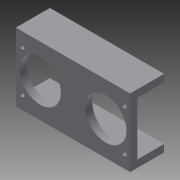
# Autodesk Inventor part: ProxSensor_Bracket
Saved by Autodesk Inventor 2015 (Build 190159000, 159)
## iProperties
Created: 2015-03-05
Part Number: ProxSensor_Bracket
Material: Generic
Document SubType Name: Modeling
Designer: ChristopherEvan
Density: 1 g/cm^3
Appearance: Default
Author: ChristopherEvan
Autodesk Inventor part; units mm, degrees
ref_plane "YZ Plane" through (0, 0, 0) normal (1, 0, 0) x (0, 1, 0)
ref_plane "XZ Plane" through (0, 0, 0) normal (0, 1, 0) x (-1, 0, 0)
ref_plane "XY Plane" through (0, 0, 0) normal (0, 0, 1) x (1, 0, 0)
sketch "Sketch1" plane through (0, 0, 0) normal (0, 0, 1) x (1, 0, 0)
  circle A0 centre (36, -10) radius 0.8353 projected
  circle A1 centre (9, -10) radius 0.8353 projected
  circle A2 centre (1.5, -1.5) radius 1 projected
  circle A3 centre (1.5, -18.5) radius 1 projected
  circle A4 centre (43.5, -1.5) radius 1 projected
  circle A5 centre (43.5, -18.5) radius 1 projected
  line L0 (0, -20) -> (45, -20) projected
  line L1 (45, -20) -> (45, 0) projected
  line L2 (45, 0) -> (0, 0) projected
  line L3 (0, 0) -> (0, -20) projected
  circle A6 centre (36, -10) radius 8.5
  line L4 (46, 1) -> (-1, 1)
  line L5 (-1, 1) -> (-1, -21)
  line L6 (-1, -21) -> (46, -21)
  line L7 (46, -21) -> (46, 1)
  circle A7 centre (9, -10) radius 8.5
  circle A8 centre (36, -10) radius 8 projected
  circle A9 centre (9, -10) radius 8 projected
  dimension "d0" = 17
  dimension "d1" = 47
  dimension "d2" = 22
  dimension "d3" = 1
  dimension "d4" = 1
  dimension "d5" = 17
  constraints: 8 end point, 2 centre point, 2 coincident, 2 parallel, 1 horizontal, 1 perpendicular
  measures "d0" diameter of A6
  measures "d1" distance between parallel lines of L5 L7
  measures "d2" distance between parallel lines of L6 L4
  measures "d3" distance between parallel lines of L1 L7
  measures "d4" distance between parallel lines of L2 L4
  measures "d5" diameter of A7
extrude "Extrusion1" add sketch "Sketch1" along normal blind 3 contours L3 L2 L1 L0 | L7 L6 L5 L4
sketch "Sketch5" plane through (46, -21, 0) normal (1, 0, 0) x (0, 0, -1)
  line L0 (-3, 0) -> (11, 0)
  line L1 (11, -3) -> (-3, -3)
  line L2 (-3, -3) -> (-3, 0)
  line L3 (11, -3) -> (14, -3)
  line L4 (14, -3) -> (14, 22)
  line L5 (14, 22) -> (11, 22)
  line L6 (11, 22) -> (11, 0)
  point P0 (0, 21)
  dimension "d12" = 3
  dimension "d14" = 3
  dimension "d15" = 22
  constraints: 14 end point, 3 parallel, 2 horizontal, 1 perpendicular
  measures "d12" distance between parallel lines of L0 L1
  measures "d14" distance between parallel lines of L6 L4
  measures "d15" distance between parallel lines of L5 L0
extrude "Extrusion2" add sketch "Sketch5" against normal blind 47
sketch "Sketch6" plane through (46, -24, -14) normal (0, 0, -1) x (-1, 0, 0)
  circle A0 centre (2.5, 22.5) radius 1 projected
  circle A1 centre (44.5, 22.5) radius 1 projected
  circle A2 centre (44.5, 5.5) radius 1 projected
  circle A3 centre (2.5, 5.5) radius 1 projected
  line L0 (0, 25) -> (47, 25) projected
  line L1 (42, 25) -> (5, 25)
  line L2 (5, 25) -> (5, 5)
  line L3 (5, 5) -> (42, 5)
  line L4 (42, 5) -> (42, 25)
  line L5 (47, 25) -> (47, 0) projected
  line L6 (0, 25) -> (0, 0) projected
  line L7 (0, 0) -> (47, 0) projected
  point P0 (46, 24)
  dimension "d18" = 5
  dimension "d19" = 5
  dimension "d20" = 5
  constraints: 8 end point, 2 parallel, 1 horizontal, 1 perpendicular, 1 point on line
  measures "d18" distance between parallel lines of L5 L4
  measures "d19" distance between parallel lines of L6 L2
  measures "d20" distance between parallel lines of L7 L3
extrude "Extrusion3" cut sketch "Sketch6" against normal up to surface (3 mm away) contours L0 L4 L3 L2
sketch "Sketch8" plane through (46, 1, -11) normal (0, 1, 0) x (1, 0, 0)
  line L0 (0, 3) -> (-47, 3)
  line L1 (-47, 3) -> (-47, -14)
  line L2 (-47, -14) -> (0, -14)
  line L3 (0, -14) -> (0, 3)
  point P0 (-46, -11)
  point P1 (0, -14)
  constraints: 8 end point, 2 parallel, 1 horizontal, 1 perpendicular
extrude "Extrusion4" add sketch "Sketch8" along normal blind 3
sketch "Sketch9" plane through (46, -24, -14) normal (0, 0, -1) x (-1, 0, 0)
  line L0 (0, 28) -> (47, 28) projected
  line L1 (0, 0) -> (0, 28) projected
  line L2 (47, 0) -> (47, 28) projected
  line L3 (0, 0) -> (47, 0) projected
  point P0 (46, 24)
extrude "Extrusion5" cut sketch "Sketch9" against normal blind 3
body "Solid1"
